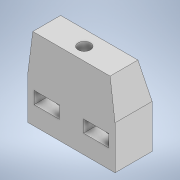
# Autodesk Inventor part: Съемная стойка сервы
Saved by Autodesk Inventor 2020 (Build 240168000, 168)
## iProperties
Created: 2021-04-19
Part Number: Съемная стойка сервы
Material: Типовые
Document SubType Name: Обычные детали
Designer: Антон
Density: 1 g/cm^3
Appearance: По умолчанию
Sheet Metal Rule: По умолчанию
Author: Антон
Autodesk Inventor part; units mm, degrees
ref_plane "YZ Plane" through (0, 0, 0) normal (1, 0, 0) x (0, 1, 0)
ref_plane "XZ Plane" through (0, 0, 0) normal (0, 1, 0) x (-1, 0, 0)
ref_plane "XY Plane" through (0, 0, 0) normal (0, 0, 1) x (1, 0, 0)
sketch "Эскиз1" plane through (0, 0, 0) normal (0, 1, 0) x (-1, 0, 0)
  line L0 (0, 0) -> (14.1, 0)
  line L1 (14.1, 0) -> (14.1, -6)
  line L2 (14.1, -6) -> (0, -6)
  line L3 (0, -6) -> (0, 0)
  dimension "d0" = 14.1
  dimension "d1" = 6
  constraints: 8 end point, 2 parallel, 1 horizontal, 1 perpendicular
  measures "d0" distance of L1.end L2.end
  measures "d1" distance of L0.end L1.end
extrude "Выдавливание1" add sketch "Эскиз1" along normal blind 13.15
sketch "Эскиз2" plane through (0, 13.15, 0) normal (0, 1, 0) x (1, 0, 0)
  line L0 (-14.1, 0) -> (0, 0) projected
  line L1 (-7.05, 0) -> (-7.05, 2.075)
  dimension "d4" = 2.075
  constraints: 2 end point, 1 midpoint, 1 vertical
  measures "d4" distance of L1.start L1.end
hole "Отверстие1" at (-7.05, 13.15, -2.075) direction (0, -1, 0) diameter 2 depth 5 tip angle 118
sketch "Эскиз3" plane through (0, 0, 0) normal (0, -1, 0) x (1, 0, 0)
  line L0 (0, 0) -> (0, -6) projected
  line L1 (0, -3) -> (-3.05, -3)
  line L2 (-14.1, -6) -> (-14.1, 0) projected
  line L3 (-14.1, -3) -> (-11.05, -3)
  line L4 (0, 0) -> (0, -6) projected
  line L5 (-14.1, -6) -> (-14.1, 0) projected
  line L6 (-14.1, 0) -> (0, 0) projected
  dimension "d12" = 3
  dimension "d24" = 8
  constraints: 4 end point, 2 collinear, 2 midpoint, 2 perpendicular
  measures "d12" distance between parallel lines of L6 L1
  measures "d24" distance of L3.end L1.end
hole "Отверстие2" at (-3.05, 0, -3) at (-11.05, 0, -3) direction (0, 1, 0) diameter 2.2 depth 5
sketch "Эскиз4" plane through (0, 0, 0) normal (0, -1, 0) x (1, 0, 0)
  circle A0 centre (-3.05, -3) radius 1.1 projected
  circle A1 centre (-11.05, -3) radius 1.1 projected
  line L0 (-3.05, -5.3671) -> (-5.1, -4.1836)
  line L1 (-5.1, -4.1836) -> (-5.1, -1.8164)
  line L2 (-5.1, -1.8164) -> (-3.05, -0.6329)
  line L3 (-3.05, -0.6329) -> (-1, -1.8164)
  line L4 (-1, -1.8164) -> (-1, -4.1836)
  line L5 (-1, -4.1836) -> (-3.05, -5.3671)
  line L6 (0, 0) -> (0, -6) projected
  line L7 (-11.05, -5.3671) -> (-13.1, -4.1836)
  line L8 (-13.1, -4.1836) -> (-13.1, -1.8164)
  line L9 (-13.1, -1.8164) -> (-11.05, -0.6329)
  line L10 (-11.05, -0.6329) -> (-9, -1.8164)
  line L11 (-9, -1.8164) -> (-9, -4.1836)
  line L12 (-9, -4.1836) -> (-11.05, -5.3671)
  line L13 (-1, -1.8164) -> (-5.1, -1.8164)
  line L14 (-5.1, -1.8164) -> (-5.1, 0)
  line L15 (-5.1, 0) -> (-1, 0)
  line L16 (-1, 0) -> (-1, -1.8164)
  line L17 (-14.1, 0) -> (0, 0) projected
  line L18 (-9, -1.8164) -> (-13.1, -1.8164)
  line L19 (-13.1, -1.8164) -> (-13.1, 0)
  line L20 (-13.1, 0) -> (-9, 0)
  line L21 (-9, 0) -> (-9, -1.8164)
  point P0 (-3.05, 0)
  point P1 (-9, 0)
  dimension "d21" = 4.1
  constraints: 40 end point, 7 parallel, 2 coincident, 2 horizontal, 2 perpendicular, 2 point on line, 1 midpoint, 26 other
  measures "d21" distance between parallel lines of L1 L4
extrude "Выдавливание2" cut sketch "Эскиз4" along normal blind 2 from surface at -5 contours A0 | A1 | L0 L1 L13 L4 L5 | L14 L15 L16 L3 L2 | L2 L3 L13 | L7 L8 L18 L11 L12 | L19 L17 L21 L10 L9 | L9 L10 L18
chamfer "Фаска1" distance 0.8 distance2 6.15 1 edges at (-14.1, 13.15, -3) measured on face at (-13.6, 13.15, -3)
chamfer "Фаска2" distance 0.8 distance2 6.15 1 edges at (0, 13.15, -3) measured on face at (-0.5, 13.15, -3)
chamfer "Фаска3" distance 1.5 distance2 6.15 1 edges at (-7.05, 13.15, -6) measured on face at (-7.05, 13.15, -5.5)
equation "\"Радиус_гибки\" = Толщина"
equation "\"Ширина_просечки\" = Толщина"
equation "\"Глубина_просечки\" = 0.5 * Толщина"
equation "\"Размер_просечки\" = 4 * Толщина"
equation "\"Мин_остаток\" = 2 * Толщина"
equation "\"Радиус_перехода\" = Радиус_гибки"
equation "\"Радиус_Якоби\" = Толщина"
equation "\"Размер_зазора\" = Толщина"
equation "\"Толщина\" = 0.5"
